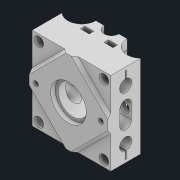
# Autodesk Inventor part: z-carriage-front
Saved by Autodesk Inventor 2021 (Build 250183000, 183)
## iProperties
Created: 2021-06-07
Part Number: z-carriage-front
Material: Generic
Document SubType Name: Modeling
Designer: arbra
Density: 1 g/cm^3
Appearance: Default
Author: arbra
Autodesk Inventor part; units mm, degrees
ref_plane "YZ Plane" through (0, 0, 0) normal (1, 0, 0) x (0, 1, 0)
ref_plane "XZ Plane" through (0, 0, 0) normal (0, 1, 0) x (-1, 0, 0)
sketch "Sketch1" plane through (0, 0, 0) normal (0, 1, 0) x (-1, 0, 0)
  line L0 (26.5, 0) -> (-26.5, 0)
  line L1 (-26.5, 0) -> (-26.5, -20.0718)
  line L2 (26.5, -20.0718) -> (26.5, 0)
  arc A0 (26.5, -20.0718) -> (10.5, -27) centre (20, -27) ccw
  arc A1 (5, -27) -> (-5, -27) centre (0, -27) ccw
  line L3 (0, -32.4) -> (0, 5.4) construction
  line L4 (-41.5779, 0) -> (41.5779, 0) construction
  arc A2 (-10.5, -27) -> (-26.5, -20.0718) centre (-20, -27) ccw
  line L5 (-10.5, -27) -> (-5, -27)
  line L6 (5, -27) -> (10.5, -27)
  line L7 (5, -27) -> (-5, -27) construction
  line L8 (-10.5, -27) -> (-26.5, -27) construction
  line L9 (-26.5, -27) -> (-26.5, -20.0718) construction
  point P0 (0, 0)
  dimension "d0" = 27
  dimension "d1" = 19
  dimension "d2" = 10
  dimension "d5" = 20
  dimension "d10" = 53
  constraints: 16 end point, 6 point on circle, 3 centre point, 3 horizontal, 3 parallel, 2 collinear, 2 perpendicular, 2 point on line, 1 midpoint, 1 symmetric about line, 2 other
  measures "d0" distance between parallel lines of L0 L5
  measures "d1" diameter of A0
  measures "d2" diameter of A1
  measures "d5" distance from line of A0.centre L3
  measures "d10" distance between parallel lines of L1 L2
extrude "Extrusion1" add sketch "Sketch1" along normal blind 56
sketch "Sketch2" plane through (-26.5, 0, 0) normal (0, 0, 1) x (1, 0, 0)
  line L0 (26.5, 57.6985) -> (-3.1985, 28)
  line L1 (-3.1985, 28) -> (26.5, -1.6985)
  line L2 (26.5, -1.6985) -> (56.1985, 28)
  line L3 (56.1985, 28) -> (26.5, 57.6985)
  line L4 (26.5, 69.5779) -> (26.5, -13.5779) construction
  line L5 (-15.0779, 0) -> (68.0779, 0) construction
  line L6 (0, 0) -> (0, 56) projected
  line L7 (0, 28) -> (53, 28) construction
  line L8 (53, 0) -> (53, 56) projected
  line L9 (0, 56) -> (53, 56) projected
  line L10 (0, 0) -> (53, 0) projected
  point P0 (24.8015, 0)
  point P1 (28.1985, 0)
  point P2 (53, 24.8015)
  point P3 (53, 31.1985)
  point P4 (28.1985, 56)
  point P5 (24.8015, 56)
  point P6 (0, 31.1985)
  point P7 (0, 24.8015)
  dimension "d8" = 42
  constraints: 10 end point, 2 midpoint, 2 parallel, 2 perpendicular, 2 point on line, 1 symmetric about line
  measures "d8" distance of L2.end L0.start
extrude "Extrusion2" add sketch "Sketch2" along normal blind 2 contours L9 L3 L8 L2 L10 L1 L6 L0
chamfer "Chamfer1" distance 2 angle 45 4 edges at (-14.0992, 43.5992, 0) (-14.0992, 12.4008, 0) (14.0992, 12.4008, 0) (14.0992, 43.5992, 0)
sketch "Sketch3" plane through (-26.5, 0, -20.0718) normal (-1, 0, 0) x (0, 0, 1)
  line L0 (10.0359, 23.125) -> (10.0359, 32.875) construction
  line L1 (14.0359, 23.125) -> (14.0359, 32.875)
  line L2 (6.0359, 32.875) -> (6.0359, 23.125)
  arc A0 (6.0359, 23.125) -> (14.0359, 23.125) centre (10.0359, 23.125) ccw
  arc A1 (14.0359, 32.875) -> (6.0359, 32.875) centre (10.0359, 32.875) ccw
  line L3 (0, 0) -> (20.0718, 0) projected
  line L4 (20.0718, 0) -> (20.0718, 21.9731) projected
  line L5 (22.0718, 24.8015) -> (20.0718, 21.9731) projected
  line L6 (22.0718, 31.1985) -> (22.0718, 24.8015) projected
  line L7 (20.0718, 34.0269) -> (22.0718, 31.1985) projected
  line L8 (20.0718, 34.0269) -> (20.0718, 56) projected
  line L9 (0, 56) -> (20.0718, 56) projected
  line L10 (0, 0) -> (0, 56) projected
  line L11 (22.0718, 31.1985) -> (20.0718, 34.0269) construction
  line L12 (20.0718, 0) -> (20.0718, 21.9731) construction
  line L13 (20.0718, 34.0269) -> (20.0718, 21.9731) construction
  line L14 (10.0359, 28) -> (20.0718, 28) construction
  line L15 (10.0359, 28) -> (0, 28) construction
  arc A2 (9.6609, 49.0828) -> (10.4109, 49.0828) centre (10.0359, 45) ccw
  line L16 (9.6609, 49.0828) -> (9.6609, 54.0828)
  line L17 (9.6609, 54.0828) -> (10.4109, 54.0828)
  line L18 (10.4109, 54.0828) -> (10.4109, 49.0828)
  line L19 (10.0359, 45) -> (10.0359, 54.0828) construction
  arc A3 (10.4109, 6.9172) -> (9.6609, 6.9172) centre (10.0359, 11) ccw
  line L20 (9.6609, 6.9172) -> (9.6609, 1.9172)
  line L21 (9.6609, 1.9172) -> (10.4109, 1.9172)
  line L22 (10.4109, 1.9172) -> (10.4109, 6.9172)
  dimension "d16" = 8
  dimension "d17" = 9.75
  dimension "d18" = 8.2
  dimension "d20" = 0.75
  dimension "d21" = 5
  dimension "d22" = 34
  constraints: 28 end point, 8 point on circle, 5 symmetric about line, 4 centre point, 4 midpoint, 4 tangent, 3 perpendicular, 3 vertical, 1 collinear, 1 horizontal, 1 parallel, 1 point on line, 2 other
  measures "d16" distance between parallel lines of L1 L2
  measures "d17" distance of L0.start L0.end
  measures "d18" diameter of A2
  measures "d20" distance of L16.end L17.end
  measures "d21" distance of L17.end L18.end
  measures "d22" distance of A3.centre L19.start
extrude "Extrusion3" cut sketch "Sketch3" against normal through all contours A0 L2 A1 L1 | L16 L17 L18 A2 | L22 L21 L20 A3
sketch "Sketch4" plane through (-26.5, 0, 2) normal (0, 0, 1) x (1, 0, 0)
  line L0 (26.5, 67.2) -> (26.5, -11.2) projected
  line L1 (0, 0) -> (0, 56) projected
  line L2 (0, 28) -> (53, 28) construction
  line L3 (53, 24.8015) -> (53, 31.1985) projected
  line L4 (26.5, 6.0797) -> (48.4203, 28)
  line L5 (48.4203, 28) -> (26.5, 49.9203)
  line L6 (26.5, 49.9203) -> (4.5797, 28)
  line L7 (4.5797, 28) -> (26.5, 6.0797)
  line L8 (26.5, 6.0797) -> (26.5, 49.9203) construction
  line L9 (48.4203, 28) -> (4.5797, 28) construction
  point P0 (26.5, 0)
  point P1 (26.5, 28)
  dimension "d123" = 31
  constraints: 14 end point, 5 midpoint, 2 coincident, 2 collinear, 2 parallel, 1 perpendicular
  measures "d123" distance of L5.end L6.end
hole "Stepper mount" at (-21.9203, 28, 2) at (21.9203, 28, 2) direction (0, 0, -1) diameter 3.3 end through all
sketch "Sketch5" plane through (-26.5, 23.125, -14.0359) normal (0, 0, 1) x (1, 0, 0)
  circle A0 centre (4.58, 4.875) radius 1.65 projected
  circle A1 centre (48.42, 4.875) radius 1.65 projected
  circle A2 centre (48.42, 4.875) radius 1.65 projected
  point P0 (26.5, -23.125)
  constraints: 2 coincident
hole "stepper mount space" at (-21.92, 28, -14.0359) at (21.92, 28, -14.0359) direction (0, 0, -1) diameter 6.4 end through all
sketch "Sketch6" plane through (-26.5, 0, 2) normal (0, 0, 1) x (1, 0, 0)
  line L0 (53, 0) -> (53, 21.9731) construction
  line L1 (0, 34.0269) -> (0, 56) construction
  line L2 (53, 0) -> (0, 56) construction
  line L3 (37, 56) -> (53, 56) construction
  line L4 (0, 0) -> (0, 21.9731) construction
  line L5 (53, 56) -> (0, 0) construction
  point P0 (26.5, 0)
  point P1 (26.5, 28)
  constraints: 4 end point, 1 midpoint
hole "Hole3" at (0, 28, 2) direction (0, 0, -1) diameter 24 depth 3
hole "Hole4" at (0, 28, 2) direction (0, 0, -1) diameter 20 depth 19
hole "Hole5" at (0, 28, 2) direction (0, 0, -1) diameter 15 end through all
sketch "Sketch7" plane through (-26.5, 56, 0) normal (0, 0, 1) x (1, 0, 0)
  line L0 (0, -21.9731) -> (0, 0) projected
  line L1 (0, 0) -> (21.9731, 0) projected
  line L2 (26.5, 11.2) -> (26.5, -67.2) construction
  circle A0 centre (4.58, -28) radius 1.65 construction
  circle A1 centre (48.42, -28) radius 1.65 construction
  line L3 (4.58, -28) -> (48.42, -28) construction
  point P0 (26.5, -56)
  point P1 (4.5, -4.5)
  point P2 (48.5, -4.5)
  point P3 (4.5, -51.5)
  point P4 (48.5, -51.5)
  dimension "d61" = 4.5
  dimension "d62" = 4.5
  constraints: 3 symmetric about line, 2 end point, 1 horizontal
  measures "d61" distance from line of point (4.5, -4.5) L0
  measures "d62" distance from line of L1 point (4.5, -4.5)
hole "Hole6" at (-22, 51.5, 0) at (22, 51.5, 0) at (-22, 4.5, 0) at (22, 4.5, 0) direction (0, 0, -1) diameter 3.3 end through all counterbore diameter 6.4 counterbore depth 4
ref_plane "Work Plane1" through (0, 0, -13.5) normal (0, 0, 1) x (1, 0, 0)
sketch "Sketch8" plane through (0, 0, -13.5) normal (0, 0, 1) x (1, 0, 0)
  circle A0 centre (-22, 51.5) radius 1.65 projected
  line L0 (-25.4641, 51.5) -> (-23.7321, 54.5)
  line L1 (-23.7321, 54.5) -> (-20.2679, 54.5)
  line L2 (-20.2679, 54.5) -> (-18.5359, 51.5)
  line L3 (-18.5359, 51.5) -> (-20.2679, 48.5)
  line L4 (-20.2679, 48.5) -> (-23.7321, 48.5)
  line L5 (-23.7321, 48.5) -> (-25.4641, 51.5)
  circle A1 centre (-22, 4.5) radius 1.65 projected
  circle A2 centre (22, 4.5) radius 1.65 projected
  line L6 (0, 67.2) -> (0, -11.2) construction
  line L7 (-37.1, 0) -> (37.1, 0) construction
  line L8 (-25.4641, 4.5) -> (-23.7321, 7.5)
  line L9 (-23.7321, 7.5) -> (-20.2679, 7.5)
  line L10 (-20.2679, 7.5) -> (-18.5359, 4.5)
  line L11 (-18.5359, 4.5) -> (-20.2679, 1.5)
  line L12 (-20.2679, 1.5) -> (-23.7321, 1.5)
  line L13 (-23.7321, 1.5) -> (-25.4641, 4.5)
  line L14 (18.5359, 51.5) -> (20.2679, 54.5)
  line L15 (20.2679, 54.5) -> (23.7321, 54.5)
  line L16 (23.7321, 54.5) -> (25.4641, 51.5)
  line L17 (25.4641, 51.5) -> (23.7321, 48.5)
  line L18 (23.7321, 48.5) -> (20.2679, 48.5)
  line L19 (20.2679, 48.5) -> (18.5359, 51.5)
  line L20 (18.5359, 4.5) -> (20.2679, 7.5)
  line L21 (20.2679, 7.5) -> (23.7321, 7.5)
  line L22 (23.7321, 7.5) -> (25.4641, 4.5)
  line L23 (25.4641, 4.5) -> (23.7321, 1.5)
  line L24 (23.7321, 1.5) -> (20.2679, 1.5)
  line L25 (20.2679, 1.5) -> (18.5359, 4.5)
  point P0 (0, 0)
  point P1 (-21.966, 3.4172)
  point P2 (-21.034, 3.4172)
  point P3 (21.034, 3.4172)
  point P4 (21.966, 3.4172)
  dimension "d71" = 6
  dimension "d72" = 47
  dimension "d73" = 44
  dimension "d76" = 47
  dimension "d79" = 44
  constraints: 48 end point, 2 horizontal, 1 coincident, 1 vertical, 51 other
  measures "d71" distance between parallel lines of L4 L1
  measures "d72" distance of point (-22, 4.5) A0.centre
  measures "d73" distance of point (22, 4.5) point (-22, 4.5)
  measures "d76" distance of L0.start L8.start
  measures "d79" distance of L0.start L14.start
extrude "Extrusion4" cut sketch "Sketch8" against normal through all contours A0 | L0 L1 L2 L3 L4 L5 | A1 | A2 | L8 L9 L10 L11 L12 L13 | L14 L15 L16 L17 L18 L19 | L20 L21 L22 L23 L24 L25
ref_plane "Work Plane2" through (0, 49.1, 0) normal (0, 1, 0) x (1, 0, 0)
sketch "Sketch12" plane through (0, 49.1, 0) normal (0, 1, 0) x (1, 0, 0)
  arc A0 (10.5, 27) -> (26.5, 20.0718) centre (20, 27) ccw construction
  arc A1 (10.5, 27) -> (18.5359, 17.6135) centre (20, 27) ccw
  line L0 (10.5, 27) -> (5, 27) projected
  line L1 (10.5, 27) -> (10.7, 27)
  line L2 (18.5359, 17.6135) -> (18.5667, 17.8111)
  arc A2 (10.7, 27) -> (18.5667, 17.8111) centre (20, 27) ccw
  line L3 (0, 32.804) -> (0, -7.8007) construction
  arc A3 (-18.5359, 17.6135) -> (-10.5, 27) centre (-20, 27) ccw
  line L4 (-10.5, 27) -> (-10.7, 27)
  line L5 (-18.5359, 17.6135) -> (-18.5667, 17.8111)
  arc A4 (-18.5667, 17.8111) -> (-10.7, 27) centre (-20, 27) ccw
  point P0 (0, 0)
  dimension "d89" = 0.2
  constraints: 8 end point, 8 point on circle, 6 symmetric about line, 4 centre point, 2 concentric, 2 line through centre, 1 equal length, 1 horizontal, 2 other
  measures "d89" distance of L0.start L1.end
extrude "Extrusion6" add sketch "Sketch12" along normal mid plane 1
ref_plane "Work Plane3" through (0, 6.9, 0) normal (0, -1, 0) x (1, 0, 0)
sketch "Sketch13" plane through (0, 6.9, 0) normal (0, -1, 0) x (1, 0, 0)
  arc A0 (18.5359, -17.6135) -> (10.5, -27) centre (20, -27) ccw projected
  line L0 (10.5, -27) -> (10.7, -27) projected
  arc A1 (18.5667, -17.8111) -> (10.7, -27) centre (20, -27) ccw projected
  line L1 (18.5667, -17.8111) -> (18.5359, -17.6135) projected
  arc A2 (-10.7, -27) -> (-18.5667, -17.8111) centre (-20, -27) ccw projected
  line L2 (-10.7, -27) -> (-10.5, -27) projected
  arc A3 (-10.5, -27) -> (-18.5359, -17.6135) centre (-20, -27) ccw projected
  line L3 (-18.5359, -17.6135) -> (-18.5667, -17.8111) projected
  point P0 (0, 0)
extrude "Extrusion7" add sketch "Sketch13" along normal mid plane 1
sketch "Sketch14" plane through (-5, 0, -27) normal (0, 0, -1) x (-1, 0, 0)
  line L0 (-5, -11.2) -> (-5, 67.2) construction
  circle A0 centre (16.92, 28) radius 1.65 projected
  circle A1 centre (-26.92, 28) radius 1.65 projected
  line L1 (16.92, 28) -> (-26.92, 28) construction
  point P0 (-5, 0)
  point P1 (3, 5.5)
  point P2 (-13, 5.5)
  point P3 (3, 50.5)
  point P4 (-13, 50.5)
  dimension "d95" = 16
  dimension "d96" = 45
  constraints: 3 symmetric about line, 2 end point, 1 horizontal
  measures "d95" distance of point (-13, 5.5) point (3, 5.5)
  measures "d96" distance of point (-13, 5.5) point (-13, 50.5)
hole "Hole7" at (-8, 5.5, -27) at (8, 5.5, -27) at (-8, 50.5, -27) at (8, 50.5, -27) direction (0, 0, 1) diameter 3.4 depth 12
ref_plane "Work Plane4" through (-5, 0, -17) normal (0, 0, -1) x (-1, 0, 0)
sketch "Sketch16" plane through (-5, 0, -17) normal (0, 0, -1) x (-1, 0, 0)
  circle A0 centre (3, 50.5) radius 1.7 construction
  line L0 (0, 46.75) -> (6, 46.75)
  line L1 (6, 46.75) -> (6, 56)
  line L2 (6, 56) -> (0, 56)
  line L3 (0, 56) -> (0, 46.75)
  line L4 (0, 56) -> (5.5, 56) projected
  line L5 (3, 50.5) -> (6, 50.5) construction
  line L6 (3, 50.5) -> (0, 50.5) construction
  line L7 (-5, -11.2) -> (-5, 67.2) construction
  circle A1 centre (-26.92, 28) radius 1.65 construction
  circle A2 centre (16.92, 28) radius 1.65 construction
  line L8 (-26.92, 28) -> (16.92, 28) construction
  line L9 (-10, 46.75) -> (-16, 46.75)
  line L10 (-16, 46.75) -> (-16, 56)
  line L11 (-16, 56) -> (-10, 56)
  line L12 (-10, 56) -> (-10, 46.75)
  line L13 (0, 9.25) -> (6, 9.25)
  line L14 (6, 9.25) -> (6, 0)
  line L15 (6, 0) -> (0, 0)
  line L16 (0, 0) -> (0, 9.25)
  line L17 (-10, 0) -> (-10, 9.25)
  line L18 (-16, 0) -> (-10, 0)
  line L19 (-16, 9.25) -> (-16, 0)
  line L20 (-10, 9.25) -> (-16, 9.25)
  point P0 (-5, 0)
  dimension "d119" = 3.75
  dimension "d120" = 6
  constraints: 38 end point, 12 symmetric about line, 3 point on line, 2 collinear, 2 horizontal, 2 parallel, 2 perpendicular
  measures "d119" distance from line of L0 L5.start
  measures "d120" distance between parallel lines of L3 L1
extrude "Extrusion9" cut sketch "Sketch16" along normal blind 3
equation "\"d62\" = d61"
equation "\"d76\" = d72"
equation "\"d79\" = d73"
body "Solid1"
